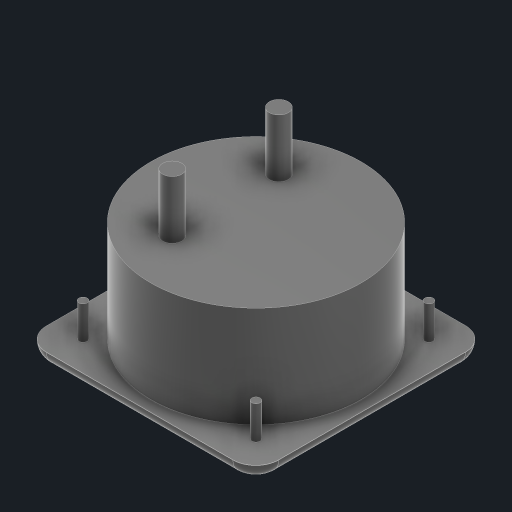
# Autodesk Inventor part: MarionEICdcAmeter
Saved by Autodesk Inventor 2024 (Build 280153000, 153)
## iProperties
Created: 2023-12-09
Part Number: MarionEICdcAmeter
Material: Acetal Resin, Black
Document SubType Name: Modeling
Designer: 16155
Density: 1.425 g/cm^3
Appearance: Smooth - Black
Author: Eli Neville
Keywords: Ammeter
Comments: This is the Ammeter I plan on using in my Multometer project.
Autodesk Inventor part; units mm, degrees
ref_plane "YZ Plane" through (0, 0, 0) normal (1, 0, 0) x (0, 1, 0)
ref_plane "XZ Plane" through (0, 0, 0) normal (0, 1, 0) x (-1, 0, 0)
ref_plane "XY Plane" through (0, 0, 0) normal (0, 0, 1) x (1, 0, 0)
sketch "Sketch1" plane through (0, 0, 0) normal (0, 1, 0) x (-1, 0, 0)
  line L0 (-38.095, 38.17) -> (38.095, 38.17)
  line L1 (38.095, 38.17) -> (38.095, -38.17)
  line L2 (38.095, -38.17) -> (-38.095, -38.17)
  line L3 (-38.095, -38.17) -> (-38.095, 38.17)
  line L4 (-38.095, 38.17) -> (38.095, -38.17) construction
  line L5 (38.095, 38.17) -> (-38.095, -38.17) construction
  line L6 (-6.095, 28.615) -> (11.095, 28.615)
  line L7 (11.095, -28.615) -> (-6.095, -28.615)
  line L8 (-11.095, -23.615) -> (-11.095, 23.615)
  line L9 (-11.095, 28.615) -> (11.095, -28.615) construction
  line L10 (11.095, 28.615) -> (-11.095, -28.615) construction
  line L11 (30.1625, 9.5) -> (30.1625, -9.5)
  arc A0 (30.1625, 9.5) -> (11.095, 28.615) centre (8.2631, 6.7226) ccw
  line L12 (38.095, 0) -> (-38.095, 0)
  arc A1 (11.095, -28.615) -> (30.1625, -9.5) centre (8.2631, -6.7226) ccw
  arc A2 (-6.095, 28.615) -> (-11.095, 23.615) centre (-6.095, 23.615) ccw
  arc A3 (-11.095, -23.615) -> (-6.095, -28.615) centre (-6.095, -23.615) ccw
  line L13 (-11.095, 0) -> (-38.095, 0)
  circle A4 centre (-24.595, 0) radius 2.89
  point P0 (0, 0)
  dimension "d0" = 76.34
  dimension "d1" = 76.19
  dimension "d2" = 57.23
  dimension "d3" = 22.19
  dimension "d5" = 5
  dimension "d6" = 5
  dimension "d7" = 5.78
  constraints: 28 end point, 8 midpoint, 8 point on circle, 5 centre point, 5 point on line, 4 tangent, 3 parallel, 2 horizontal, 1 collinear, 1 perpendicular, 1 symmetric about line, 1 other
  measures "d0" distance of L0.end L1.end
  measures "d1" distance of L1.end L2.end
  measures "d2" distance of L6.end L7.start
  measures "d3" distance of L7.start L10.end
  measures "d5" radius of A2
  measures "d6" radius of A3
  measures "d7" diameter of A4
extrude "Extrusion1" add sketch "Sketch1" along normal blind 5 contours L0 L1 L12 L11 A0 L6 A2 L8 A4 L3 | L12 A4 L8 A3 L7 A1 L11 L1 L2 L3
sketch "Sketch2" plane through (0, 5, 0) normal (0, 1, 0) x (1, 0, 0)
  circle A0 centre (0, 0) radius 34.5
  dimension "d10" = 69
  constraints: 1 centre point, 1 coincident
  measures "d10" diameter of A0
extrude "Extrusion2" add sketch "Sketch2" along normal blind 33.12
sketch "Sketch3" plane through (0, 5, 0) normal (0, 1, 0) x (1, 0, 0)
  line L0 (28.385, 28.385) -> (-28.385, 28.385)
  line L1 (-28.385, 28.385) -> (-28.385, -28.385)
  line L2 (-28.385, -28.385) -> (28.385, -28.385)
  line L3 (28.385, -28.385) -> (28.385, 28.385)
  line L4 (28.385, 28.385) -> (-28.385, -28.385) construction
  line L5 (-28.385, 28.385) -> (28.385, -28.385) construction
  circle A0 centre (28.385, -28.385) radius 1.375
  circle A1 centre (-28.385, 28.385) radius 1.375
  circle A2 centre (-28.385, -28.385) radius 1.375
  circle A3 centre (28.385, 28.385) radius 1.375
  point P0 (0, 0)
  dimension "d13" = 56.77
  dimension "d14" = 56.77
  dimension "d15" = 2.75
  dimension "d16" = 2.75
  dimension "d18" = 2.75
  dimension "d19" = 2.75
  constraints: 12 end point, 4 centre point, 4 coincident, 2 midpoint, 2 parallel, 1 horizontal, 1 perpendicular
  measures "d13" distance of L1.end L2.end
  measures "d14" distance of L0.end L1.end
  measures "d15" diameter of A0
  measures "d16" diameter of A3
  measures "d18" diameter of A1
  measures "d19" diameter of A2
extrude "Extrusion3" add sketch "Sketch3" along normal blind 10.9 contours A1 L1 L0 | L0 L1 A1 | A3 L3 L0 | L0 L3 A3 | A2 L2 L1 | L1 L2 A2 | A0 L2 L3 | L3 L2 A0
sketch "Sketch5" plane through (0, 38.12, 0) normal (0, 1, 0) x (1, 0, 0)
  line L0 (10, 17.5) -> (-10, 17.5)
  line L1 (-10, 17.5) -> (-10, -17.5)
  line L2 (-10, -17.5) -> (10, -17.5)
  line L3 (10, -17.5) -> (10, 17.5)
  line L4 (10, 17.5) -> (-10, -17.5) construction
  line L5 (-10, 17.5) -> (10, -17.5) construction
  circle A0 centre (-10, 17.5) radius 3.125
  circle A1 centre (-10, -17.5) radius 3.125
  point P0 (0, 0)
  dimension "d32" = 35
  dimension "d33" = 20
  dimension "d34" = 6.25
  dimension "d35" = 6.25
  constraints: 12 end point, 2 centre point, 2 coincident, 2 midpoint, 2 parallel, 1 horizontal, 1 perpendicular, 1 point on line
  measures "d32" distance of L0.end L1.end
  measures "d33" distance of L0.start L0.end
  measures "d34" diameter of A0
  measures "d35" diameter of A1
extrude "Extrusion5" add sketch "Sketch5" along normal blind 19 contours A0 L1 L0 | L0 L1 A0 | A1 L1 L2 | L2 L1 A1
fillet "Fillet1" radius 7.5 4 edges at (-38.095, 2.5, 38.17) (38.095, 2.5, 38.17) (38.095, 2.5, -38.17) (-38.095, 2.5, -38.17)
fillet "Fillet2" radius 4.9 8 edges at (-35.8983, 0, -35.9733) (-38.095, 0, 0) (-35.8983, 0, 35.9733) (0, 0, 38.17) (35.8983, 0, 35.9733) (38.095, 0, 0) (35.8983, 0, -35.9733) (0, 0, -38.17)
body "Solid1"
